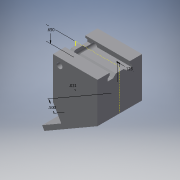
# Autodesk Inventor part: Gantry_Mount
Saved by Autodesk Inventor 2019 (Build 230136000, 136)
## iProperties
Created: 2021-01-31
Part Number: Gantry_Mount
Material: Generic
Document SubType Name: Modeling
Designer: zhanb
Density: 1 g/cm^3
Appearance: Default
Author: zhanb
Autodesk Inventor part; units mm, degrees
ref_plane "YZ Plane" through (0, 0, 0) normal (1, 0, 0) x (0, 1, 0)
ref_plane "XZ Plane" through (0, 0, 0) normal (0, 1, 0) x (-1, 0, 0)
ref_plane "XY Plane" through (0, 0, 0) normal (0, 0, 1) x (1, 0, 0)
sketch "Sketch1" plane through (0, 0, 0) normal (0, 0, 1) x (1, 0, 0)
  line L0 (-25.4, -35.56) -> (-18.5941, -35.56) construction
  line L1 (25.4, -35.56) -> (25.4, -10.16) construction
  line L2 (25.4, 35.56) -> (-25.4, 35.56)
  line L3 (-25.4, 35.56) -> (-25.4, -33.6235)
  line L4 (-25.4, -35.56) -> (25.4, 35.56) construction
  line L5 (25.4, -35.56) -> (-25.4, 35.56) construction
  line L6 (-18.5941, -35.56) -> (25.4, -10.16)
  line L7 (-18.5941, -35.56) -> (-35.0919, -45.085)
  line L8 (-35.0919, -45.085) -> (-37.6319, -40.6856)
  line L9 (-37.6319, -40.6856) -> (-25.4, -33.6235)
  line L10 (-21.1341, -31.1606) -> (-18.5941, -35.56) construction
  line L11 (-18.5941, -35.56) -> (25.4, -35.56) construction
  line L12 (-25.4, -33.6235) -> (-25.4, -35.56) construction
  line L13 (-25.4, -33.6235) -> (-21.1341, -31.1606) construction
  line L14 (25.4, -10.16) -> (25.4, 35.56)
  point P0 (0, 0)
  dimension "d0" = 30
  dimension "d1" = 50.8
  dimension "d2" = 71.12
  dimension "d3" = 50.8
  dimension "d4" = 5.08
  dimension "d5" = 19.05
  constraints: 30 end point, 9 parallel, 5 perpendicular, 2 horizontal, 2 midpoint, 1 point on line
  measures "d0" angle of L0 L6
  measures "d1" distance of L0.end L1.end
  measures "d2" distance of L2.end L0.start
  measures "d3" distance of L2.start L2.end
  measures "d4" distance of L7.end L8.end
  measures "d5" distance of L0.end L7.end
extrude "Extrusion1" add sketch "Sketch1" along normal mid plane 50.8
sketch "Sketch3" plane through (0, 0, 0) normal (0, 0, 1) x (1, 0, 0)
  line L0 (25.4, 35.56) -> (-25.4, 35.56) construction
  line L1 (-25.4, 35.56) -> (-25.4, -33.6235) construction
  line L2 (-25.4, -33.6235) -> (-37.6319, -40.6856) construction
  line L3 (-37.6319, -40.6856) -> (-35.0919, -45.085) construction
  line L4 (-35.0919, -45.085) -> (25.4, -10.16) construction
  line L5 (25.4, -10.16) -> (25.4, 35.56) construction
  line L6 (-25.4, 19.05) -> (7.6889, 19.05)
  line L7 (22.225, 19.05) -> (22.225, 14.4034) construction
  line L8 (22.225, -6.1272) -> (-15.8226, -28.094)
  line L9 (-25.4, -33.6235) -> (-25.4, 35.56) construction
  line L10 (-25.4, 19.05) -> (-25.4, -11.5054)
  line L11 (22.225, 8.5375) -> (15.875, 4.8713) construction
  line L12 (-22.1726, -17.0955) -> (-24.7126, -12.6961)
  line L13 (-24.7126, -12.6961) -> (13.335, 9.2707)
  line L14 (22.225, 14.4034) -> (22.225, 19.05) construction
  line L15 (25.4, -10.16) -> (25.4, 35.56) construction
  line L16 (22.225, 8.5375) -> (22.225, -6.1272) construction
  line L17 (22.225, 14.4034) -> (22.225, 8.5375) construction
  line L18 (22.225, -6.1272) -> (15.875, 4.8713)
  line L19 (13.335, 9.2707) -> (7.6889, 19.05)
  line L20 (13.335, 9.2707) -> (22.225, 14.4034) construction
  line L21 (15.875, 4.8713) -> (-22.1726, -17.0955)
  line L22 (7.6889, 19.05) -> (22.225, 19.05) construction
  line L23 (-24.7126, -12.6961) -> (-25.4, -11.5054)
  line L24 (-25.4, 35.56) -> (-25.4, -33.6235) projected
  line L25 (-22.1726, -17.0955) -> (-15.8226, -28.094)
  line L26 (-25.4, -11.5054) -> (-25.4, -33.6235)
  line L27 (-15.8226, -28.094) -> (-25.4, -33.6235)
  point P0 (0, 0)
  point P1 (-25.4, -13.0929)
  dimension "d8" = 16.51
  dimension "d9" = 3.175
  dimension "d45" = 12.7
  dimension "d50" = 0.7937
  constraints: 38 end point, 12 perpendicular, 7 point on line, 4 parallel, 2 horizontal, 2 vertical, 1 collinear
  measures "d8" distance between parallel lines of L0 L6
  measures "d9" distance between parallel lines of L5 L7
  measures "d45" distance between parallel lines of L2 L11
  measures "d50" distance of point (-25.4, -13.093) L12.end
extrude "Extrusion2" cut sketch "Sketch3" along normal mid plane 40.64 contours L6 L19 L13 L23 L10 | L21 L18 L8 L25
sketch "Sketch5" plane through (-25.4, -33.6235, 25.4) normal (-1, 0, 0) x (0, 0, 1)
  line L0 (-50.8, 0) -> (0, 0) construction
  line L1 (0, 69.1835) -> (0, 0) construction
  line L2 (-50.8, 69.1835) -> (0, 69.1835) construction
  line L3 (-50.8, 0) -> (-50.8, 69.1835) construction
  line L4 (-36.83, 69.1835) -> (-36.83, 66.842)
  line L5 (-36.83, 66.842) -> (-39.37, 64.302)
  line L6 (-39.37, 64.302) -> (-39.37, 61.762)
  line L7 (-39.37, 61.762) -> (-33.02, 61.762)
  line L8 (-33.02, 61.762) -> (-29.845, 64.937)
  line L9 (-29.845, 64.937) -> (-20.955, 64.937)
  line L10 (-20.955, 64.937) -> (-17.78, 61.762)
  line L11 (-17.78, 61.762) -> (-11.43, 61.762)
  line L12 (-11.43, 61.762) -> (-11.43, 64.302)
  line L13 (-11.43, 64.302) -> (-13.97, 66.842)
  line L14 (-13.97, 66.842) -> (-13.97, 69.1835)
  line L15 (-45.72, 52.6735) -> (-5.08, 52.6735) projected
  line L16 (-25.4, 52.6735) -> (-25.4, 69.1835) construction
  line L17 (-36.83, 69.1835) -> (-13.97, 69.1835)
  point P0 (-25.4, 33.6235)
  dimension "d22" = 135
  dimension "d23" = 11.43
  dimension "d24" = 2.3416
  dimension "d25" = 2.54
  dimension "d26" = 3.175
  dimension "d27" = 13.97
  dimension "d28" = 6.35
  constraints: 26 end point, 4 parallel, 4 point on line, 2 midpoint, 2 perpendicular, 1 collinear, 5 other
  measures "d22" angle of L8 L9
  measures "d23" distance between parallel lines of L16 L4
  measures "d24" distance of L4.start L4.end
  measures "d25" distance of L5.end L6.end
  measures "d26" distance between parallel lines of L7 L9
  measures "d27" distance between parallel lines of L16 L6
  measures "d28" distance of L6.end L7.end
extrude "Extrusion3" cut sketch "Sketch5" against normal through all
sketch "Sketch6" plane through (0, 0, 25.4) normal (0, 0, 1) x (1, 0, 0)
  line L0 (-25.4, 28.1384) -> (25.4, 28.1384) construction
  line L1 (-25.4, 28.1384) -> (25.4, 28.1384) construction
  circle A0 centre (-17.78, 28.0495) radius 3.2639
  line L2 (-25.4, 35.56) -> (-25.4, -33.6235) projected
  line L3 (25.4, 35.56) -> (-25.4, 35.56) projected
  line L4 (-25.4, 31.3134) -> (25.4, 31.3134) construction
  point P0 (0, 0)
  point P1 (0, 28.1384)
  dimension "d32" = 6.5278
  dimension "d35" = 7.62
  dimension "d39" = 3.2639
  constraints: 1 centre point, 1 coincident, 1 midpoint
  measures "d32" diameter of A0
  measures "d35" distance from line of L2 A0.centre
  measures "d39" distance from line of L4 point (-17.78, 28.05)
extrude "Extrusion4" cut sketch "Sketch6" against normal through all
sketch "Sketch7" plane through (0, 0, 0) normal (0, 0, 1) x (1, 0, 0)
  circle A0 centre (-17.78, 28.0495) radius 3.2639 construction
  arc A1 (-19.7144, 30.6784) -> (-21.0427, 28.1384) centre (-17.78, 28.0495) ccw construction
  line L0 (-21.0439, 28.0495) -> (-21.0439, 31.3134)
  line L1 (-21.0439, 31.3134) -> (-14.5161, 31.3134)
  line L2 (-14.5161, 31.3134) -> (-14.5161, 28.0495)
  arc A2 (-21.0427, 28.1384) -> (-15.8456, 30.6784) centre (-17.78, 28.0495) ccw construction
  arc A3 (-21.0439, 28.0495) -> (-14.5161, 28.0495) centre (-17.78, 28.0495) ccw
  point P0 (0, 0)
  point P1 (-25.4, 31.3134)
  constraints: 6 end point, 4 point on circle, 3 tangent, 1 centre point, 1 coincident, 1 horizontal alignment, 1 parallel, 1 perpendicular, 1 vertical
extrude "Extrusion5" cut sketch "Sketch7" along normal up to surface (22.86 mm away) from surface at -11.43
sketch "Sketch8" plane through (25.4, -10.16, -25.4) normal (0.5, -0.8660254, 0) x (0.8660254, 0.5, 0)
  circle A0 centre (-25.4, 25.4) radius 14.3129
  line L0 (0, 0) -> (0, 50.8) construction
  line L1 (-69.85, 50.8) -> (0, 50.8) construction
  line L2 (-69.85, 0) -> (-69.85, 50.8) construction
  line L3 (0, 0) -> (-69.85, 0) construction
  line L4 (0, 50.8) -> (-50.8, 0) construction
  line L5 (-55.7258, 0) -> (-21.1341, 0) construction
  point P0 (-16.917, 25.4)
  dimension "d40" = 28.6258
  dimension "d41" = 45
  constraints: 2 end point, 1 centre point, 1 coincident, 1 midpoint, 1 point on line
  measures "d40" diameter of A0
  measures "d41" angle of L1 L4
extrude "Extrusion6" cut sketch "Sketch8" against normal up to surface (22.86 mm away)
extrude "Extrusion7" cut sketch "Sketch3" along normal through all both and the other way through all contours L23 L12 L25 L27 L24
equation "\"d39\" = 0.5 * d32"
body "Solid1"
